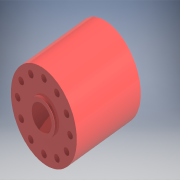
# Autodesk Inventor part: shaft
Saved by Autodesk Inventor 2018 (Build 220112000, 112)
## iProperties
Created: 2023-12-05
Part Number: shaft
Material: Steel
Document SubType Name: Modeling
Designer: DDUGKY
Density: 7.85 g/cm^3
Appearance: Default
Author: DDUGKY
Autodesk Inventor part; units mm, degrees
ref_plane "YZ Plane" through (0, 0, 0) normal (1, 0, 0) x (0, 1, 0)
ref_plane "XZ Plane" through (0, 0, 0) normal (0, 1, 0) x (-1, 0, 0)
ref_plane "XY Plane" through (0, 0, 0) normal (0, 0, 1) x (1, 0, 0)
sketch "Sketch1" plane through (0, 0, 0) normal (0, 0, 1) x (1, 0, 0)
  circle A0 centre (0, 0) radius 30
  dimension "d0" = 60
  constraints: 1 centre point, 1 coincident
  measures "d0" diameter of A0
extrude "Extrusion1" add sketch "Sketch1" along normal mid plane 58.037
sketch "Sketch2" plane through (0, 0, 0) normal (0, 0, 1) x (1, 0, 0)
  circle A0 centre (0, 0) radius 30 projected
  circle A1 centre (0, 0) radius 12
  dimension "d3" = 24
  constraints: 1 centre point, 1 coincident
  measures "d3" diameter of A1
extrude "Extrusion2" add sketch "Sketch2" along normal mid plane 62.037 contours A1
sketch "Sketch3" plane through (0, 0, 0) normal (0, 0, 1) x (1, 0, 0)
  circle A0 centre (0, 0) radius 12 projected
  circle A1 centre (0, 0) radius 9
  dimension "d6" = 18
  constraints: 1 centre point, 1 coincident
  measures "d6" diameter of A1
extrude "Extrusion3" cut sketch "Sketch3" along normal mid plane 94.75 contours A1
sketch "Sketch4" plane through (0, 0, 0) normal (0, 0, 1) x (1, 0, 0)
  circle A0 centre (0, 0) radius 23.75
  circle A1 centre (0, 23.75) radius 2.5
  dimension "d9" = 47.5
  dimension "d10" = 5
  constraints: 1 centre point, 1 coincident, 1 vertical alignment, 2 other
  measures "d10" diameter of A1
extrude "Extrusion4" cut sketch "Sketch4" along normal mid plane 127.5 contours A1 A0 | A0 A1 picked at (-0.0971, 22.9126) picked at (0.0803, 24.5697)
pattern_circular "Circular Pattern1" count 12 over 360 about axis through (0, 0, 0) along (0, 0, 1) of "Extrusion4"
body "Solid1"
